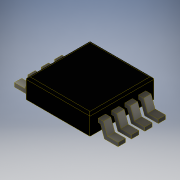
# Autodesk Inventor part: uMax8
Saved by Autodesk Inventor 2016 (Build 200138000, 138)
## iProperties
Created: 2016-09-14
Part Number: uMax8
Material: Generic
Document SubType Name: Modeling
Designer: jfixelle
Density: 1 g/cm^3
Appearance: Silver
Author: jfixelle
Autodesk Inventor part; units mm, degrees
ref_plane "YZ Plane" through (0, 0, 0) normal (1, 0, 0) x (0, 1, 0)
ref_plane "XZ Plane" through (0, 0, 0) normal (0, 1, 0) x (-1, 0, 0)
sketch "Sketch1" plane through (0, 0, 0) normal (0, 1, 0) x (-1, 0, 0)
  line L0 (1.55, 1.55) -> (-1.55, 1.55)
  line L1 (-1.55, 1.55) -> (-1.55, -1.55)
  line L2 (-1.55, -1.55) -> (1.55, -1.55)
  line L3 (1.55, -1.55) -> (1.55, 1.55)
  point P0 (0, 0)
  dimension "d0" = 3.1
  dimension "d1" = 1.55
  dimension "d2" = 3.1
  dimension "d3" = 1.55
  constraints: 8 end point, 2 parallel, 1 horizontal, 1 perpendicular
  measures "d0" distance of L2.end L0.start
  measures "d1" distance from line of L2 point (0, 0)
  measures "d2" distance of L1.end L2.end
  measures "d3" distance from line of point (0, 0) L3
extrude "Extrusion1" add sketch "Sketch1" along normal blind 0.95
fillet "Fillet1" radius 0.1 4 edges at (0, 0.95, 1.55) (1.55, 0.95, 0) (0, 0.95, -1.55) (-1.55, 0.95, 0)
ref_plane "Work Plane1" through (0, 0, 0.325) normal (0, 0, 1) x (1, 0, 0)
sketch "Sketch2" plane through (0, 0, 0.325) normal (0, 0, 1) x (1, 0, 0)
  line L0 (1.8068, 0.565) -> (1.319, 0.565)
  line L1 (1.319, 0.565) -> (1.319, 0.385)
  line L2 (1.319, 0.385) -> (1.6603, 0.385)
  line L3 (1.6603, 0.385) -> (1.855, -0.15)
  line L4 (1.855, -0.15) -> (2.515, -0.15)
  line L5 (2.515, -0.15) -> (2.515, 0.03)
  line L6 (2.515, 0.03) -> (2.0015, 0.03)
  line L7 (2.0015, 0.03) -> (1.8068, 0.565)
  line L8 (-1.55, 0) -> (1.55, 0) projected
  line L9 (0, 0) -> (0, -0.2043)
  dimension "d8" = 0.15
  dimension "d9" = 2.515
  dimension "d10" = 0.66
  dimension "d11" = 0.18
  dimension "d12" = 0.18
  dimension "d13" = 0.565
  dimension "d15" = 70
  dimension "d16" = 70
  constraints: 18 end point, 4 perpendicular, 1 horizontal, 1 parallel, 1 vertical
  measures "d8" distance between parallel lines of L4 L8
  measures "d9" distance between parallel lines of L5 L9
  measures "d10" distance of L3.end L4.end
  measures "d11" distance of L4.end L5.end
  measures "d12" distance between parallel lines of L2 L0
  measures "d13" distance between parallel lines of L8 L0
  measures "d15" angle of L7 L6
  measures "d16" angle of L4 L3
extrude "Extrusion2" add sketch "Sketch2" along normal mid plane 0.36
pattern_linear "Rectangular Pattern1" count 4 spacing 0.65 along (0, 0, -1) of "Extrusion2" first direction both ways yes
mirror "Mirror1" about plane through (0, 0, 0) normal (1, 0, 0) of "Extrusion2", "Rectangular Pattern1"
body "Solid1"
